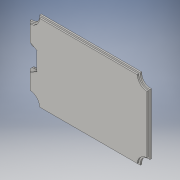
# Autodesk Inventor part: battbase__lid_final
Saved by Autodesk Inventor 2016 (Build 200138000, 138)
## iProperties
Created: 2016-06-18
Part Number: battbase__lid_final
Material: Generic
Document SubType Name: Modeling
Designer: jsharp
Density: 1 g/cm^3
Appearance: Default
Author: jsharp
Autodesk Inventor part; units mm, degrees
ref_plane "YZ Plane" through (0, 0, 0) normal (1, 0, 0) x (0, 1, 0)
ref_plane "XZ Plane" through (0, 0, 0) normal (0, 1, 0) x (-1, 0, 0)
ref_plane "XY Plane" through (0, 0, 0) normal (0, 0, 1) x (1, 0, 0)
sketch "Sketch1" plane through (0, 0, 0) normal (0, 0, 1) x (1, 0, 0)
  line L0 (-43.5443, 19.427) -> (49.4557, 19.427)
  line L1 (52.4557, 16.427) -> (52.4557, -43.573)
  line L2 (49.4557, -46.573) -> (-43.5443, -46.573)
  line L3 (-46.5443, -43.573) -> (-46.5443, 16.427)
  arc A0 (-43.5443, 19.427) -> (-46.5443, 16.427) centre (-43.5443, 16.427) ccw
  arc A1 (-46.5443, -43.573) -> (-43.5443, -46.573) centre (-43.5443, -43.573) ccw
  arc A2 (49.4557, -46.573) -> (52.4557, -43.573) centre (49.4557, -43.573) ccw
  arc A3 (52.4557, 16.427) -> (49.4557, 19.427) centre (49.4557, 16.427) ccw
  point P0 (0, 0)
  point P1 (0, 0)
  point P2 (-46.5443, 19.427)
  point P3 (52.4557, -46.573)
  point P4 (52.4557, 19.427)
  dimension "d0" = 99
  dimension "d1" = 66
  dimension "d2" = 3
  constraints: 8 end point, 8 point on circle, 8 tangent, 6 point on line, 4 centre point, 3 equal radius, 2 parallel, 1 horizontal, 1 perpendicular
  measures "d0" distance of point (-46.544, 19.427) point (52.456, 19.427)
  measures "d1" distance of point (52.456, 19.427) point (52.456, -46.573)
  measures "d2" radius of A0
extrude "Extrusion1" add sketch "Sketch1" along normal blind 1.27
sketch "Sketch2" plane through (0, 0, 1.27) normal (0, 0, 1) x (1, 0, 0)
  line L0 (-46.5443, 16.427) -> (-46.5443, -43.573) projected
  line L1 (49.4557, 19.427) -> (-43.5443, 19.427) projected
  circle A0 centre (-42.7343, 15.617) radius 1.5875
  line L2 (-50.0562, -13.573) -> (79.0191, -13.573) construction
  line L3 (2.9557, 30.2203) -> (2.9557, -48.7988) construction
  circle A1 centre (-42.7343, -42.763) radius 1.5875
  circle A2 centre (48.6457, 15.617) radius 1.5875
  circle A3 centre (48.6457, -42.763) radius 1.5875
  point P0 (0, 0)
  dimension "d8" = 3.175
  dimension "d9" = 3.81
  dimension "d10" = 3.81
  constraints: 4 centre point, 4 end point, 3 symmetric about line, 1 horizontal, 1 vertical, 3 other
  measures "d8" diameter of A0
  measures "d9" distance from line of L1 A0.centre
  measures "d10" distance from line of L0 A0.centre
extrude "Extrusion2" cut sketch "Sketch2" against normal blind 25.4
sketch "Sketch3" plane through (0, 0, 1.27) normal (0, 0, 1) x (1, 0, 0)
  circle A0 centre (48.6457, 15.617) radius 1.5875 projected
  circle A1 centre (-42.7343, 15.617) radius 1.5875 projected
  circle A2 centre (-42.7343, -42.763) radius 1.5875 projected
  circle A3 centre (48.6457, -42.763) radius 1.5875 projected
  line L0 (49.4557, 19.427) -> (-43.5443, 19.427) projected
  arc A4 (-43.5443, 19.427) -> (-46.5443, 16.427) centre (-43.5443, 16.427) ccw projected
  line L1 (-46.5443, 16.427) -> (-46.5443, -43.573) construction
  arc A5 (-46.5443, -43.573) -> (-43.5443, -46.573) centre (-43.5443, -43.573) ccw projected
  line L2 (-43.5443, -46.573) -> (49.4557, -46.573) projected
  arc A6 (49.4557, -46.573) -> (52.4557, -43.573) centre (49.4557, -43.573) ccw projected
  line L3 (52.4557, -43.573) -> (52.4557, 16.427) projected
  arc A7 (52.4557, 16.427) -> (49.4557, 19.427) centre (49.4557, 16.427) ccw projected
  arc A8 (-43.5443, 19.427) -> (-46.5443, 16.427) centre (-43.5443, 16.427) ccw projected
  line L4 (49.4557, 19.427) -> (-43.5443, 19.427) projected
  circle A9 centre (48.6457, 15.617) radius 1.5875 projected
  circle A10 centre (-42.7343, 15.617) radius 1.5875 projected
  circle A11 centre (-42.7343, -42.763) radius 1.5875 projected
  circle A12 centre (48.6457, -42.763) radius 1.5875 projected
  arc A13 (52.4557, 16.427) -> (49.4557, 19.427) centre (49.4557, 16.427) ccw projected
  line L5 (52.4557, 16.427) -> (52.4557, -43.573) projected
  arc A14 (49.4557, -46.573) -> (52.4557, -43.573) centre (49.4557, -43.573) ccw projected
  line L6 (49.4557, -46.573) -> (-43.5443, -46.573) projected
  arc A15 (-46.5443, -43.573) -> (-43.5443, -46.573) centre (-43.5443, -43.573) ccw projected
  line L7 (-46.5443, -43.573) -> (-46.5443, 16.427) projected
  arc A16 (-43.5443, 19.427) -> (-46.5443, 16.427) centre (-43.5443, 16.427) ccw projected
  line L8 (-43.5443, 19.427) -> (49.4557, 19.427) projected
  line L9 (-43.5443, 19.427) -> (49.4557, 19.427) projected
  line L10 (-40.8039, 19.427) -> (-40.8039, -46.573) construction
  line L11 (49.4557, -46.573) -> (-43.5443, -46.573) projected
  line L12 (-40.8039, 19.427) -> (-51.3078, 19.427) construction
  line L13 (-40.8039, -46.573) -> (-51.3078, -46.573) construction
  line L14 (-40.8039, -21.173) -> (-51.3078, -21.173) construction
  line L15 (-40.8039, -5.973) -> (-51.3078, -5.973) construction
  line L16 (-46.5443, -43.573) -> (-46.5443, 16.427) projected
  line L17 (-46.5443, -5.973) -> (-40.8039, -5.973)
  line L18 (-40.8039, -5.973) -> (-40.8039, -21.173)
  line L19 (-40.8039, -21.173) -> (-46.5443, -21.173)
  line L20 (-46.5443, -21.173) -> (-46.5443, -5.973)
  point P0 (0, 0)
  dimension "d13" = 25.4
  dimension "d14" = 25.4
  dimension "d15" = 5.7404
  constraints: 18 end point, 7 point on line, 4 horizontal, 2 parallel, 2 perpendicular
  measures "d13" distance between parallel lines of L13 L14
  measures "d14" distance between parallel lines of L15 L12
  measures "d15" distance between parallel lines of L10 L1
extrude "Extrusion3" cut sketch "Sketch3" against normal blind 25.4 contours L17 L18 L19 L7
fillet "Fillet1" radius 3.175 2 edges at (-46.5443, -21.173, 0.635) (-46.5443, -5.973, 0.635)
sketch "Sketch9" plane through (0, 0, 1.27) normal (0, 0, 1) x (1, 0, 0)
  arc A0 (-43.5443, 19.427) -> (-46.5443, 16.427) centre (-43.5443, 16.427) ccw projected
  line L0 (-46.5443, -2.798) -> (-46.5443, 16.427) construction
  line L1 (-46.5443, 16.427) -> (-46.5443, -2.798)
  line L2 (-43.5443, 19.427) -> (-26.5771, 19.427) construction
  line L3 (49.4557, 19.427) -> (-43.5443, 19.427) projected
  line L4 (-45.6657, 18.5483) -> (-26.5771, -0.5403) construction
  line L5 (-45.6657, 18.5483) -> (-18.6704, 18.5483) construction
  circle A1 centre (-45.6657, 18.5483) radius 7.1603
  arc A2 (-46.5443, -2.798) -> (-43.3693, -5.973) centre (-43.3693, -2.798) ccw projected
  line L6 (-43.3693, -5.973) -> (-40.8039, -5.973) projected
  line L7 (-40.8039, -5.973) -> (-40.8039, -21.173) projected
  line L8 (-40.8039, -21.173) -> (-43.3693, -21.173) projected
  arc A3 (-43.3693, -21.173) -> (-46.5443, -24.348) centre (-43.3693, -24.348) ccw projected
  line L9 (-46.5443, -24.348) -> (-46.5443, -43.573) projected
  arc A4 (-46.5443, -43.573) -> (-43.5443, -46.573) centre (-43.5443, -43.573) ccw projected
  line L10 (-43.5443, -46.573) -> (49.4557, -46.573) projected
  arc A5 (49.4557, -46.573) -> (52.4557, -43.573) centre (49.4557, -43.573) ccw projected
  line L11 (52.4557, -43.573) -> (52.4557, 16.427) projected
  arc A6 (52.4557, 16.427) -> (49.4557, 19.427) centre (49.4557, 16.427) ccw projected
  line L12 (49.4557, 19.427) -> (-43.5443, 19.427) projected
  arc A7 (-43.5443, 19.427) -> (-46.5443, 16.427) centre (-43.5443, 16.427) ccw projected
  line L13 (-46.5443, 16.427) -> (-46.5443, -2.798) projected
  circle A8 centre (48.6457, 15.617) radius 1.5875 projected
  circle A9 centre (-42.7343, 15.617) radius 1.5875 projected
  circle A10 centre (-42.7343, -42.763) radius 1.5875 projected
  circle A11 centre (48.6457, -42.763) radius 1.5875 projected
  line L14 (-75.7777, -13.573) -> (114.1059, -13.573) construction
  line L15 (2.9557, 31.1348) -> (2.9557, -53.319) construction
  circle A12 centre (-45.6657, -45.6944) radius 7.1603
  line L16 (2.9557, -58.2809) -> (2.9557, 26.1729) construction
  circle A13 centre (51.577, 18.5483) radius 7.1603
  circle A14 centre (51.577, -45.6944) radius 7.1603
  point P0 (0, 0)
  dimension "d28" = 45
  constraints: 14 end point, 5 symmetric about line, 4 centre point, 2 horizontal, 2 vertical, 1 coincident, 1 equal length, 1 point on circle, 1 point on line, 1 tangent, 3 other
  measures "d28" angle of L4 L5
extrude "Extrusion5" cut sketch "Sketch9" against normal blind 12.7 contours L3 A1 L1 A0 | A0 L1 A1 L3 | A13 L11 A6 L3 | L3 A6 L11 A13 | A14 L10 A5 L11 | L11 A5 L10 A14 | A12 L9 A4 L10 | L10 A4 L9 A12
sketch "Sketch10" plane through (0, 0, 1.27) normal (0, 0, 1) x (1, 0, 0)
  arc A0 (52.4557, -38.5882) -> (44.4708, -46.573) centre (51.577, -45.6944) ccw projected
  line L0 (52.4557, -38.5882) -> (52.4557, 11.4421) projected
  arc A1 (44.4708, 19.427) -> (52.4557, 11.4421) centre (51.577, 18.5483) ccw projected
  line L1 (44.4708, 19.427) -> (-38.5595, 19.427) projected
  arc A2 (-46.5443, 11.4421) -> (-38.5595, 19.427) centre (-45.6657, 18.5483) ccw projected
  line L2 (-46.5443, 11.4421) -> (-46.5443, -2.798) projected
  arc A3 (-46.5443, -2.798) -> (-43.3693, -5.973) centre (-43.3693, -2.798) ccw projected
  line L3 (-43.3693, -5.973) -> (-40.8039, -5.973) projected
  line L4 (-40.8039, -5.973) -> (-40.8039, -21.173) projected
  line L5 (-40.8039, -21.173) -> (-43.3693, -21.173) projected
  arc A4 (-43.3693, -21.173) -> (-46.5443, -24.348) centre (-43.3693, -24.348) ccw projected
  line L6 (-46.5443, -24.348) -> (-46.5443, -38.5882) projected
  arc A5 (-38.5595, -46.573) -> (-46.5443, -38.5882) centre (-45.6657, -45.6944) ccw projected
  line L7 (-38.5595, -46.573) -> (44.4708, -46.573) projected
  line L8 (-36.7645, -45.303) -> (43.1467, -45.303)
  line L9 (-36.7645, 18.157) -> (43.1467, 18.157)
  line L10 (44.4708, 19.427) -> (-38.5595, 19.427) projected
  line L11 (-36.7645, -45.303) -> (-37.2353, -45.303)
  arc A6 (-38.5595, -46.573) -> (-46.5443, -38.5882) centre (-45.6657, -45.6944) ccw projected
  line L12 (-36.7645, 18.157) -> (-37.2353, 18.157)
  line L13 (51.1857, 10.118) -> (51.1857, -37.264)
  arc A7 (44.4708, 19.427) -> (52.4557, 11.4421) centre (51.577, 18.5483) ccw projected
  line L14 (-39.5339, -5.973) -> (-39.5339, -21.173)
  line L15 (-45.2743, -2.798) -> (-39.5339, -5.973)
  line L16 (-39.5339, -21.173) -> (-45.2743, -24.348)
  line L17 (51.1857, 10.118) -> (52.4557, 10.118) construction
  line L18 (52.4557, -38.5882) -> (52.4557, 11.4421) projected
  line L19 (43.1467, 18.157) -> (43.1467, 19.427) construction
  arc A8 (43.1467, 18.157) -> (51.1857, 10.118) centre (51.577, 18.5483) ccw
  line L20 (-56.5649, -13.573) -> (80.9191, -13.573) construction
  line L21 (2.9557, 34.2968) -> (2.9557, -68.6615) construction
  arc A9 (51.1857, -37.264) -> (43.1467, -45.303) centre (51.577, -45.6944) ccw
  arc A10 (-45.2743, 10.118) -> (-37.2353, 18.157) centre (-45.6657, 18.5483) ccw
  arc A11 (-37.2353, -45.303) -> (-45.2743, -37.264) centre (-45.6657, -45.6944) ccw
  line L22 (-45.2743, 10.118) -> (-45.2743, -2.798)
  line L23 (-45.2743, -37.264) -> (-45.2743, -24.348)
  line L24 (-46.5443, -43.573) -> (-46.5443, -24.348) projected
  point P0 (0, 0)
  dimension "d31" = 1.27
  dimension "d32" = 1.27
  dimension "d35" = 1.27
  dimension "d36" = 1.27
  dimension "d39" = 3.175
  dimension "d40" = 3.175
  dimension "d42" = 1.27
  dimension "d43" = 1.27
  dimension "d44" = 1.2791
  constraints: 28 end point, 9 symmetric about line, 8 point on circle, 4 centre point, 4 parallel, 3 vertical, 2 perpendicular, 2 point on line, 1 horizontal, 3 other
  measures "d31" distance between parallel lines of L9 L1
  measures "d32" distance between parallel lines of L7 L8
  measures "d35" distance between parallel lines of L0 L13
  measures "d36" distance between parallel lines of L14 L4
  measures "d39" vertical distance of L14.end L16.end
  measures "d40" vertical distance of L15.start L14.start
  measures "d42" distance edge to line of A1 L17
  measures "d43" distance edge to line of A1 L19
  measures "d44" radial gap between concentric circles of A8 A1
extrude "Extrusion6" cut sketch "Sketch10" against normal blind 7.62 contours L11 A11 L23 L16 L14 L15 L22 A10 L12 L9 A8 L13 A9 L8
sketch "Sketch13" plane through (0, 0, 1.27) normal (0, 0, 1) x (1, 0, 0)
  arc A0 (51.1857, -37.264) -> (43.1467, -45.303) centre (51.577, -45.6944) ccw projected
  line L0 (43.1467, -45.303) -> (-37.2353, -45.303) projected
  arc A1 (-37.2353, -45.303) -> (-45.2743, -37.264) centre (-45.6657, -45.6944) ccw projected
  line L1 (-45.2743, -37.264) -> (-45.2743, -24.348) projected
  line L2 (-45.2743, -24.348) -> (-39.5339, -21.173) projected
  line L3 (-39.5339, -21.173) -> (-39.5339, -5.973) projected
  line L4 (-39.5339, -5.973) -> (-45.2743, -2.798) projected
  line L5 (-45.2743, -2.798) -> (-45.2743, 10.118) projected
  arc A2 (-45.2743, 10.118) -> (-37.2353, 18.157) centre (-45.6657, 18.5483) ccw projected
  line L6 (-37.2353, 18.157) -> (43.1467, 18.157) projected
  arc A3 (43.1467, 18.157) -> (51.1857, 10.118) centre (51.577, 18.5483) ccw projected
  line L7 (51.1857, 10.118) -> (51.1857, -37.264) projected
  arc A4 (52.4557, -38.5882) -> (44.4708, -46.573) centre (51.577, -45.6944) ccw projected
  line L8 (52.4557, -38.5882) -> (52.4557, 11.4421) projected
  arc A5 (44.4708, 19.427) -> (52.4557, 11.4421) centre (51.577, 18.5483) ccw projected
  line L9 (44.4708, 19.427) -> (-38.5595, 19.427) projected
  arc A6 (-46.5443, 11.4421) -> (-38.5595, 19.427) centre (-45.6657, 18.5483) ccw projected
  line L10 (-46.5443, 11.4421) -> (-46.5443, -2.798) projected
  arc A7 (-46.5443, -2.798) -> (-43.3693, -5.973) centre (-43.3693, -2.798) ccw projected
  line L11 (-43.3693, -5.973) -> (-40.8039, -5.973) projected
  line L12 (-40.8039, -5.973) -> (-40.8039, -21.173) projected
  line L13 (-40.8039, -21.173) -> (-43.3693, -21.173) projected
  arc A8 (-43.3693, -21.173) -> (-46.5443, -24.348) centre (-43.3693, -24.348) ccw projected
  line L14 (-46.5443, -24.348) -> (-46.5443, -38.5882) projected
  arc A9 (-38.5595, -46.573) -> (-46.5443, -38.5882) centre (-45.6657, -45.6944) ccw projected
  line L15 (-38.5595, -46.573) -> (44.4708, -46.573) projected
  point P0 (0, 0)
extrude "Extrusion9" add sketch "Sketch13" along normal blind 1.27 and the other way blind 1.27 contours A0 L0 A1 L1 L2 L3 L4 L5 A2 L6 A3 L7
body "Solid1"
